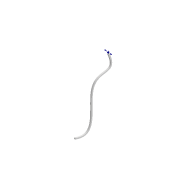
# Autodesk Inventor part: Fiber_test
Saved by Autodesk Inventor 2022.5 (Build 265521000, 521)
## iProperties
Created: 2024-03-12
Part Number: Fiber_test
Material: Generic
Document SubType Name: Modeling
Designer: wanghaoran
Density: 1 g/cm^3
Appearance: Default
Author: wanghaoran
Autodesk Inventor part; units mm, degrees
ref_plane "YZ Plane" through (0, 0, 0) normal (1, 0, 0) x (0, 1, 0)
ref_plane "XZ Plane" through (0, 0, 0) normal (0, 1, 0) x (-1, 0, 0)
ref_plane "XY Plane" through (0, 0, 0) normal (0, 0, 1) x (1, 0, 0)
sketch "Sketch1" plane through (0, 0, 0) normal (1, 0, 0) x (0, 1, 0)
  circle A0 centre (-47.1976, 27.8404) radius 2 projected
  spline S0 degree 4 poles (0, 0) (-33.7196, -15.0107) (22.4041, 44.5208) (-60.9637, -9.0907) (-47.1976, 27.8404) knots 0 0 0 0 0 1 1 1 1 1
  line L0 (-47.1976, 27.8404) -> (-46.2606, 27.4912)
  line L1 (-0.4067, 0.9136) -> (0, 0)
  spline S1 degree 5 poles (-0.4067, 0.9136) (-1.4832, 0.4349) (-2.5714, -0.0181) (-3.6763, -0.428) (-5.3908, -0.9887) (-7.1678, -1.2886) (-7.7831, -1.3478) (-8.7513, -1.3498) (-9.6539, -1.037) (-9.95, -0.8759) (-10.4772, -0.4117) (-10.8241, 0.1965) (-10.967, 0.5326) (-11.2406, 1.3209) (-11.4195, 2.1375) (-11.5061, 2.5996) (-11.6705, 3.5793) (-11.8238, 4.5604) (-11.9086, 5.0763) (-12.1, 6.1153) (-12.3545, 7.1409) (-12.5049, 7.6535) (-12.8625, 8.6658) (-13.3483, 9.6231) (-13.6287, 10.085) (-14.2809, 10.9788) (-15.0788, 11.7461) (-15.5223, 12.1004) (-16.5161, 12.7661) (-17.6028, 13.2683) (-18.1921, 13.491) (-19.4856, 13.8958) (-20.8149, 14.163) (-21.5322, 14.2753) (-23.0759, 14.4631) (-24.628, 14.56) (-25.4566, 14.5931) (-27.1926, 14.6331) (-28.9292, 14.6296) (-29.8365, 14.621) (-31.6763, 14.5984) (-33.5163, 14.5822) (-34.4489, 14.5801) (-36.2669, 14.5976) (-38.0828, 14.682) (-38.9661, 14.7452) (-40.6046, 14.9164) (-42.2205, 15.2388) (-42.958, 15.4285) (-44.2776, 15.8765) (-45.473, 16.5843) (-45.9753, 16.9693) (-46.9079, 17.9764) (-47.4243, 19.2567) (-47.5676, 19.9836) (-47.7247, 21.9599) (-47.3843, 23.9309) (-47.0784, 25.135) (-46.6951, 26.3249) (-46.2606, 27.4912) knots 0 0 0 0 0 0 0.088018 0.088018 0.088018 0.134306 0.134306 0.134306 0.158821 0.158821 0.158821 0.185964 0.185964 0.185964 0.221114 0.221114 0.221114 0.260165 0.260165 0.260165 0.300016 0.300016 0.300016 0.340201 0.340201 0.340201 0.382379 0.382379 0.382379 0.429323 0.429323 0.429323 0.483518 0.483518 0.483518 0.545455 0.545455 0.545455 0.613244 0.613244 0.613244 0.68292 0.68292 0.68292 0.749044 0.749044 0.749044 0.805873 0.805873 0.805873 0.852444 0.852444 0.852444 0.906958 0.906958 0.906958 1 1 1 1 1 1
  point P0 (-12.3692, 1.8393)
  point P1 (-15.2528, 10.4894)
  point P2 (-34.3094, 13.5861)
  dimension "d1" = 1
  constraints: 4 end point, 8 other
sketch "Sketch2" plane through (0, 0, 0) normal (0, 1, 0) x (-1, 0, 0)
  circle A0 centre (0, 0) radius 0.5
  dimension "d0" = 1
  constraints: 1 centre point, 1 coincident
  measures "d0" diameter of A0
extrude "Extrusion1" add sketch "Sketch1" along normal blind 1 contours S0 L0 S1 A0 | A0 S1 L1 S0 picked at (-46.7567, 27.0699)
body "Solid1"
